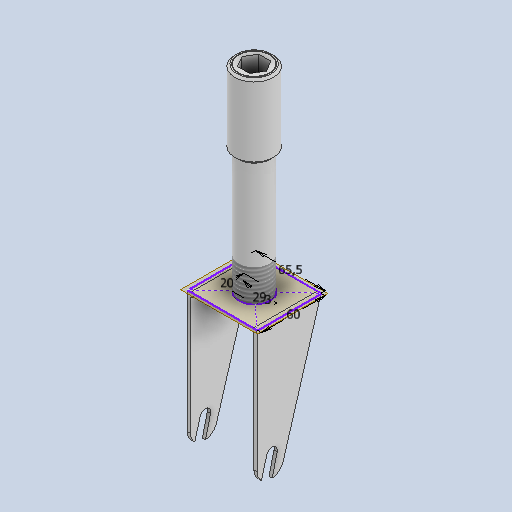
# Autodesk Inventor part: frontwheelFork
Saved by Autodesk Inventor 2022.2 (Build 262287000, 287)
## iProperties
Created: 2022-04-06
Part Number: frontwheelFork
Material: Generic
Document SubType Name: Modeling
Designer: Finn Oriwohl
Density: 1 g/cm^3
Appearance: Default
Author: Finn Oriwohl
Autodesk Inventor part; units mm, degrees
ref_plane "YZ Plane" through (0, 0, 0) normal (1, 0, 0) x (0, 1, 0)
ref_plane "XZ Plane" through (0, 0, 0) normal (0, 1, 0) x (-1, 0, 0)
ref_plane "XY Plane" through (0, 0, 0) normal (0, 0, 1) x (1, 0, 0)
sketch "Sketch1" plane through (0, 0, 0) normal (0, 1, 0) x (-1, 0, 0)
  line L0 (32.75, 30) -> (-32.75, 30)
  line L1 (-32.75, 30) -> (-32.75, -30)
  line L2 (-32.75, -30) -> (32.75, -30)
  line L3 (32.75, -30) -> (32.75, 30)
  line L4 (32.75, 30) -> (-32.75, -30) construction
  line L5 (-32.75, 30) -> (32.75, -30) construction
  line L6 (-5.7735, -10) -> (-11.547, 0)
  line L7 (-11.547, 0) -> (-5.7735, 10)
  line L8 (-5.7735, 10) -> (5.7735, 10)
  line L9 (5.7735, 10) -> (11.547, 0)
  line L10 (11.547, 0) -> (5.7735, -10)
  line L11 (5.7735, -10) -> (-5.7735, -10)
  circle A0 centre (0, 0) radius 14.5
  circle A1 centre (0, 0) radius 11.5
  point P0 (0, 10)
  point P1 (11.4997, -0.0819)
  point P2 (5.8208, -9.9181)
  point P3 (5.6789, -10)
  point P4 (-5.6789, -10)
  point P5 (-5.8208, -9.9181)
  point P6 (-11.4997, -0.0819)
  point P7 (-11.4997, 0.0819)
  point P8 (-5.8208, 9.9181)
  point P9 (-5.6789, 10)
  point P10 (5.6789, 10)
  point P11 (5.8208, 9.9181)
  point P12 (11.4997, 0.0819)
  dimension "d1" = 65.5
  dimension "d2" = 60
  dimension "d3" = 20
  dimension "d31" = 29
  dimension "d32" = 3
  constraints: 24 end point, 3 midpoint, 2 centre point, 2 parallel, 1 coincident, 1 horizontal, 1 perpendicular, 13 other
  measures "d1" distance of L2.end L1.end
  measures "d2" distance of L1.end L0.end
  measures "d3" distance from line of L11 point (0, 10)
  measures "d31" diameter of A0
  measures "d32" radial gap between concentric circles of A0 A1
extrude "Extrusion1" add sketch "Sketch1" against normal blind 3 contours L3 L2 L1 L0 | L6 A1 L11 | A1 L6 | L6 A1 L7 L8 L9 L10 L11 | L11 A1 | L6 L7 A1 | A1 L10 L11 | A1 L7 | L10 A1 | L7 L8 A1 | A1 L9 L10 | A1 L8 | L8 L9 A1 | L9 A1 | A0
ref_plane "Work Plane1" through (0, -3, 0) normal (0, -1, 0) x (1, 0, 0)
sketch "Sketch3" plane through (0, -3, 0) normal (0, -1, 0) x (1, 0, 0)
  line L0 (32.75, -30) -> (32.75, 30) projected
  line L1 (32.75, 30) -> (-32.75, 30) projected
  line L2 (-32.75, 30) -> (-32.75, -30) projected
  line L3 (-32.75, -30) -> (32.75, -30) projected
  line L4 (29.75, 30) -> (29.75, -30)
  line L5 (0, 0) -> (0, -7) construction
  line L6 (-29.75, 30) -> (-29.75, -30)
  dimension "d13" = 3
  constraints: 6 end point, 2 point on line, 2 symmetric about line, 1 perpendicular, 1 vertical
  measures "d13" distance between parallel lines of L0 L4
extrude "Extrusion4" add sketch "Sketch3" along normal blind 127 contours L3 L4 L1 L0 | L3 L2 L1 L6
sketch "Sketch4" plane through (32.75, 0, 30) normal (1, 0, 0) x (0, 0, -1)
  line L0 (0, 0) -> (60, 0) projected
  line L1 (0, 0) -> (0, -130) projected
  line L2 (60, -130) -> (0, -130) projected
  line L3 (60, 0) -> (60, -130) projected
  line L4 (0, 0) -> (60, 0) projected
  line L5 (60, 0) -> (21.1215, -130)
  arc A0 (18.8567, -108.1886) -> (9.1837, -105.6571) centre (14, -107) ccw
  line L6 (14, -107) -> (28, -107) construction
  line L7 (0, 0) -> (0, -130) projected
  line L8 (9.1837, -105.6571) -> (2, -131.4205)
  line L9 (2, -131.4205) -> (12.5394, -134)
  line L10 (12.5394, -134) -> (18.8567, -108.1886)
  arc A1 (0, -114.9326) -> (24.5531, -118.5255) centre (12.5394, -114.9326) ccw
  point P0 (30, 0)
  point P1 (14.163, -127.3665)
  point P2 (4.0294, -124.1422)
  point P3 (2.3961, -130)
  point P4 (13.5184, -130)
  dimension "d16" = 130
  dimension "d18" = 10
  dimension "d19" = 107
  dimension "d20" = 14
  dimension "d23" = 14
  constraints: 10 end point, 4 point on circle, 4 point on line, 4 tangent, 2 centre point, 1 horizontal
  measures "d16" distance between parallel lines of L2 L0
  measures "d18" diameter of A0
  measures "d19" distance from line of L0 L6.start
  measures "d20" distance of L6.start L6.end
  measures "d23" distance from line of L1 L6.start
extrude "Extrusion5" cut sketch "Sketch4" against normal blind 127 contours L3 L2 L5 | A1 L8 L2 L1 | L5 L2 L10 A1 | A1 L10 L2 L8 | L8 A0 L10 A1 | L2 L10 L9 L8
extrude "Extrusion6" add sketch "Sketch1" along normal blind 185 contours L6 A1 L11 | A1 L6 | L11 A1 | L6 L7 A1 | A1 L10 L11 | A1 L7 | L10 A1 | L7 L8 A1 | A1 L9 L10 | A1 L8 | L8 L9 A1 | L9 A1 | A0
sketch "Sketch5" plane through (0, 185, 0) normal (0, 1, 0) x (1, 0, 0)
  circle A0 centre (0, 0) radius 15
  circle A1 centre (0, 0) radius 18.1
  circle A2 centre (0, 0) radius 14.5 projected
  dimension "d35" = 36.2
  dimension "d36" = 0.5
  constraints: 2 centre point, 2 coincident
  measures "d35" diameter of A1
  measures "d36" radial gap between concentric circles of A2 A0
extrude "Extrusion7" add sketch "Sketch5" against normal blind 70 contours A1
chamfer "Chamfer1" distance 2 angle 45 1 edges at (-18.1, 185, 0)
chamfer "Chamfer2" distance 3 angle 45 1 edges at (-18.1, 115, 0)
thread "Thread3" size "M30x3.5" class "6g" standard "ANSI Metric M Profile" length 30
fillet "Fillet1" radius 2.5 2 edges at (-29.75, -3, 0.4486) (29.75, -3, 0.4486)
fillet "Fillet2" radius 3.5 2 edges at (-32.75, 0, 0) (32.75, 0, 0)
ref_plane "Work Plane2" through (32.75, 0, 30) normal (0, 1, 0) x (0, 0, -1)
split body "Split1" result two bodies by plane through (32.75, 0, 30) normal (0, 1, 0) first body at (-13.8187, 123.3333, -2.2458) (17.5429, 139.6667, 1.4162)
equation "\"d23\" = d20"
body "Solid2"
body "Solid3"
